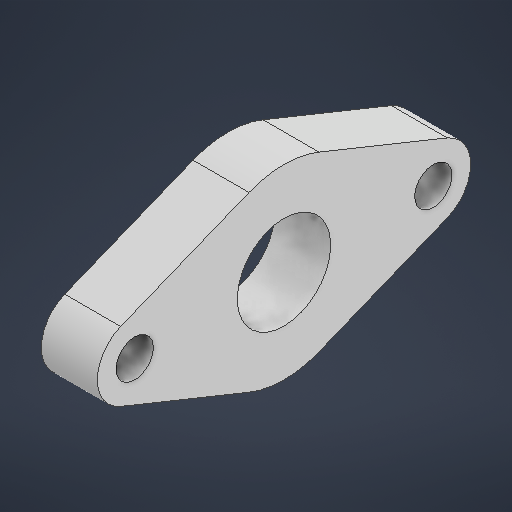
# Autodesk Inventor part: Part3
Saved by Autodesk Inventor 2026 (Build 300175050, 175E)
## iProperties
Created: 2026-03-26
Part Number: Part3
Material: Generic
Document SubType Name: Modeling
Designer: Administrator
Density: 1 g/cm^3
Appearance: Default
Author: Administrator
Autodesk Inventor part; units mm, degrees
ref_plane "YZ Plane" through (0, 0, 0) normal (1, 0, 0) x (0, 1, 0)
ref_plane "XZ Plane" through (0, 0, 0) normal (0, 1, 0) x (-1, 0, 0)
ref_plane "XY Plane" through (0, 0, 0) normal (0, 0, 1) x (1, 0, 0)
sketch "Sketch1" plane through (0, 0, 0) normal (1, 0, 0) x (0, 1, 0)
  line L0 (0, 0) -> (0, -80) construction
  line L1 (0, -80) -> (0, -40) construction
  circle A0 centre (0, 0) radius 5
  circle A1 centre (0, -80) radius 5
  circle A2 centre (0, -40) radius 12.5
  arc A3 (9.2702, 3.75) -> (-9.2702, 3.75) centre (0, 0) ccw
  arc A4 (-9.2702, -83.75) -> (9.2702, -83.75) centre (0, -80) ccw
  line L2 (23.1756, -30.625) -> (9.2702, 3.75)
  line L3 (9.2702, -83.75) -> (23.1756, -49.375)
  line L4 (26.968, -40) -> (26.9992, -39.9228)
  line L5 (-9.2702, 3.75) -> (-23.1756, -30.625)
  line L6 (-23.1756, -49.375) -> (-9.2702, -83.75)
  arc A5 (23.1756, -49.375) -> (23.1756, -30.625) centre (0, -40) ccw
  arc A6 (-23.1756, -30.625) -> (-23.1756, -49.375) centre (0, -40) ccw
  dimension "d0" = 80
  dimension "d1" = 40
  dimension "d2" = 10
  dimension "d3" = 10
  dimension "d4" = 25
  dimension "d6" = 20
  dimension "d7" = 20
  constraints: 14 end point, 10 tangent, 8 point on circle, 7 centre point, 6 coincident, 1 midpoint, 1 vertical
  measures "d0" distance of L0.start L0.end
  measures "d1" distance of L0.end L1.end
  measures "d2" diameter of A0
  measures "d3" diameter of A1
  measures "d4" diameter of A2
  measures "d6" diameter of A3
  measures "d7" diameter of A4
extrude "Extrusion1" add sketch "Sketch1" along normal mid plane 15
body "Solid1"
